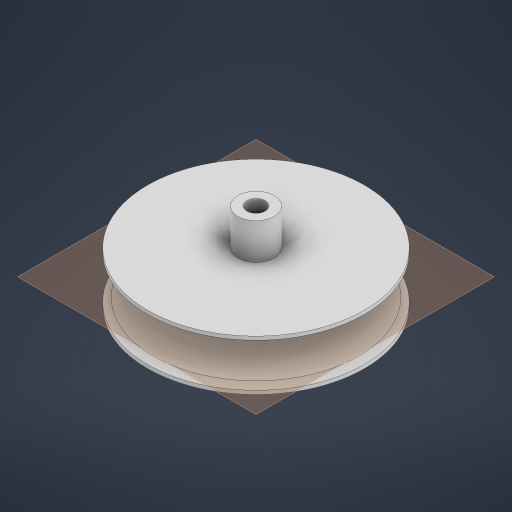
# Autodesk Inventor part: spool
Saved by Autodesk Inventor 2024 (Build 280153000, 153)
## iProperties
Created: 2026-03-23
Part Number: spool
Material: Generic
Document SubType Name: Modeling
Designer: schar
Density: 1 g/cm^3
Appearance: Default
Author: schar
Autodesk Inventor part; units mm, degrees
ref_plane "YZ Plane" through (0, 0, 0) normal (1, 0, 0) x (0, 1, 0)
ref_plane "XZ Plane" through (0, 0, 0) normal (0, 1, 0) x (-1, 0, 0)
ref_plane "XY Plane" through (0, 0, 0) normal (0, 0, 1) x (1, 0, 0)
sketch "Sketch1" plane through (0, 0, 0) normal (0, 1, 0) x (-1, 0, 0)
  circle A0 centre (0, 0) radius 30
  circle A1 centre (0, 0) radius 2.5
  dimension "d0" = 60
  dimension "d1" = 5
  constraints: 2 centre point, 2 coincident
  measures "d0" diameter of A0
  measures "d1" diameter of A1
extrude "Extrusion1" add sketch "Sketch1" along normal blind 2
sketch "Sketch2" plane through (0, 2, 0) normal (0, 1, 0) x (1, 0, 0)
  circle A0 centre (0, 0) radius 2.5
  circle A1 centre (0, 0) radius 6.5
  dimension "d4" = 13
  constraints: 2 centre point, 2 coincident
  measures "d4" diameter of A1
extrude "Extrusion2" add sketch "Sketch2" along normal blind 10
sketch "Sketch3" plane through (0, 12, 0) normal (0, 1, 0) x (1, 0, 0)
  circle A0 centre (0, 0) radius 30
  circle A1 centre (0, 0) radius 2.5
  constraints: 2 centre point, 2 coincident
extrude "Extrusion3" add sketch "Sketch3" along normal blind 2
sketch "Sketch4" plane through (0, 0, 0) normal (1, 0, 0) x (0, 1, 0)
  line L0 (2, 6.5) -> (12, 6.5) projected
  line L1 (2, 6.5) -> (3.5, 6.5)
  line L2 (2, -30) -> (2, 30) projected
  line L3 (3.5, 6.5) -> (2, 30)
  line L4 (12, 6.5) -> (10.5, 6.5)
  line L5 (12, -30) -> (12, 30) projected
  line L6 (10.5, 6.5) -> (12, 30)
  line L7 (-2.8, 0) -> (16.8, 0) projected
  point P0 (0, 0)
  dimension "d9" = 1.5
  dimension "d10" = 1.5
  constraints: 8 end point, 3 point on line
  measures "d9" distance of L1.start L1.end
  measures "d10" distance of L0.end L4.end
revolve "Revolution1" add sketch "Sketch4" angle 360 about axis through (0, -10, 0) along (0, 1, 0) contours L2 L3 L0 | L6 L5 L0
sketch "Sketch6" plane through (0, 0, 0) normal (1, 0, 0) x (0, 1, 0)
  line L0 (0, -30) -> (0, 30) projected
  line L1 (0, 30) -> (1, 30)
  line L2 (0, 30) -> (2, 30) projected
  line L3 (1, 30) -> (2.1063, 28.3339)
  line L4 (2, 30) -> (3.5, 6.5) projected
  line L5 (2.1063, 28.3339) -> (1, 28.3339)
  line L6 (1, 28.3339) -> (1, 30)
  line L7 (14, -30) -> (14, 30) projected
  line L8 (14, 30) -> (13, 30)
  line L9 (12, 30) -> (14, 30) projected
  line L10 (13, 30) -> (11.8937, 28.3339)
  line L11 (10.5, 6.5) -> (12, 30) projected
  line L12 (11.8937, 28.3339) -> (14, 28.3339)
  line L13 (14, 28.3339) -> (14, 30)
  line L14 (13, 30) -> (13, 28.3339)
  line L15 (-2.8, 0) -> (16.8, 0) projected
  point P0 (0, 0)
  dimension "d12" = 1
  dimension "d13" = 2
  constraints: 18 end point, 4 perpendicular, 4 point on line, 2 midpoint, 1 collinear
  measures "d12" distance of L0.end L1.end
  measures "d13" distance of L1.end L3.end
revolve "Revolution2" cut sketch "Sketch6" angle 360 about axis through (0, -10, 0) along (0, 1, 0) contours L2 L4 L3 | L10 L11 L9
sketch "Sketch7" plane through (0, 14, 0) normal (0, 1, 0) x (1, 0, 0)
  circle A0 centre (0, 0) radius 2.5
  circle A1 centre (0, 0) radius 5
  dimension "d15" = 10
  constraints: 2 centre point, 2 coincident
  measures "d15" diameter of A1
extrude "Extrusion4" add sketch "Sketch7" along normal blind 10
ref_plane "Work Plane1" through (0, 7, 0) normal (0, 1, 0) x (1, 0, 0)
sketch "Sketch8" plane through (0, 0, 0) normal (0, -1, 0) x (1, 0, 0)
  line L0 (0, 0) -> (8, 0)
  circle A0 centre (8, 0) radius 1
  circle A1 centre (6.9282, 4) radius 1
  dimension "d18" = 8
  dimension "d21" = 30
  dimension "d25" = 2
  constraints: 2 centre point, 2 end point, 1 coincident, 1 horizontal, 3 other
  measures "d18" distance of L0.start L0.end
  measures "d25" diameter of A0
extrude "Extrusion5" cut sketch "Sketch8" against normal up to surface
body "Solid1"
